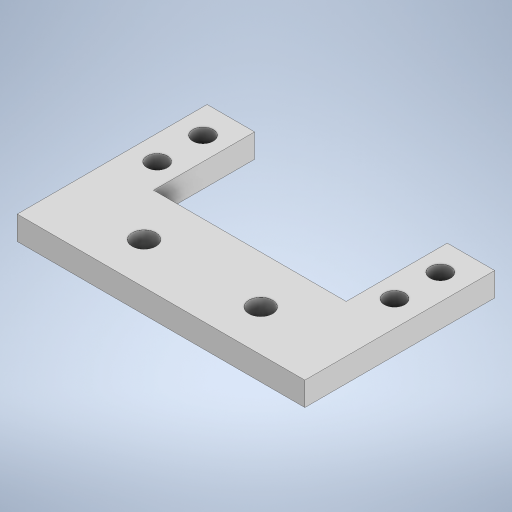
# Autodesk Inventor part: mieng_do_servo_5mm
Saved by Autodesk Inventor 2023 (Build 270158000, 158)
## iProperties
Created: 2022-11-20
Part Number: mieng_do_servo_5mm
Material: Generic
Document SubType Name: Modeling
Designer: ADMIN
Density: 1 g/cm^3
Appearance: Default
Author: ADMIN
Autodesk Inventor part; units mm, degrees
ref_plane "YZ Plane" through (0, 0, 0) normal (1, 0, 0) x (0, 1, 0)
ref_plane "XZ Plane" through (0, 0, 0) normal (0, 1, 0) x (-1, 0, 0)
ref_plane "XY Plane" through (0, 0, 0) normal (0, 0, 1) x (1, 0, 0)
sketch "Sketch1" plane through (0, 0, 0) normal (0, 1, 0) x (-1, 0, 0)
  circle A0 centre (42.9, 4.825) radius 2.15
  circle A1 centre (42.9, -4.825) radius 2.15
  circle A2 centre (-7.1, 4.825) radius 2.15
  circle A3 centre (-7.1, -4.825) radius 2.15
  line L0 (-2.4829, 9.9) -> (-2.4829, -10.8967)
  line L1 (-2.4829, -10.8967) -> (-12.4829, -10.8967)
  line L2 (-12.4829, -10.8967) -> (-12.4829, 29.1033)
  line L3 (38.1036, 9.8612) -> (38.1036, -10.8967)
  line L4 (38.1036, -10.8967) -> (48.1036, -10.8967)
  line L5 (48.1036, -10.8967) -> (48.1036, 29.1033)
  line L6 (48.1036, 29.1033) -> (-12.4829, 29.1033)
  line L7 (37.8, 10.3955) -> (-2.4829, 10.3955)
  line L8 (37.8, 10.3955) -> (38.1036, 10.3955)
  line L9 (38.1036, 10.3955) -> (38.1036, 9.8612)
  line L10 (-2.4829, 10.3955) -> (-2.4829, 9.9)
  circle A4 centre (30.1036, 20.3955) radius 2.5
  circle A5 centre (5.5171, 20.3955) radius 2.5
  point P0 (0, 0)
  point P1 (17.9, 0)
  point P2 (44.6821, 6.0277)
  point P3 (44.6821, -3.6223)
  point P4 (43.1036, -10.8967)
  dimension "d10" = 4.3
  dimension "d11" = 4.3
  dimension "d0" = 10
  dimension "d1" = 40
  dimension "d2" = 10
  dimension "d3" = 40
  dimension "d4" = 5
  dimension "d5" = 5
  dimension "d6" = 18
  dimension "d7" = 18
  dimension "d8" = 10
  dimension "d9" = 10
  dimension "d12" = 4.3
  dimension "d13" = 4.3
  dimension "d14" = 4.7964
  dimension "d15" = 4.7964
  dimension "d16" = 9.65
  dimension "d17" = 6.0717
  dimension "d18" = 9.65
  dimension "d19" = 6.0717
  dimension "d20" = 4.6171
  dimension "d21" = 4.6171
  constraints: 22 end point, 4 centre point, 4 perpendicular, 3 horizontal, 3 vertical, 1 midpoint, 1 parallel, 6 other
  measures "d0" distance of L0.end L1.end
  measures "d1" distance of L1.end L6.end
  measures "d2" distance of L3.end L5.start
  measures "d3" distance of L5.start L5.end
  measures "d4" diameter of A4
  measures "d5" diameter of A5
  measures "d6" distance from line of L5 A4.centre
  measures "d7" distance from line of A5.centre L2
  measures "d8" distance from line of L7 A4.centre
  measures "d9" distance from line of L7 A5.centre
  measures "d12" diameter of A3
  measures "d13" diameter of A2
  measures "d14" distance from line of L3 point (42.9, 4.825)
  measures "d15" distance from line of L3 point (42.9, -4.825)
  measures "d16" distance of point (42.9, -4.825) point (42.9, 4.825)
  measures "d17" vertical distance of point (43.104, -10.897) point (42.9, -4.825)
  measures "d18" distance of A3.centre A2.centre
  measures "d19" distance from line of L1 A3.centre
  measures "d20" distance from line of L0 A2.centre
  measures "d21" distance from line of L0 A3.centre
extrude "Extrusion1" add sketch "Sketch1" along normal blind 5
body "Solid1"
